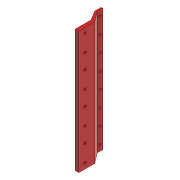
# Autodesk Inventor part: intake guide mount
Saved by Autodesk Inventor 2020 (Build 240168000, 168)
## iProperties
Created: 2020-02-10
Part Number: intake guide mount
Material: Generic
Document SubType Name: Modeling
Designer: ball
Density: 1 g/cm^3
Appearance: Default
Author: ball
Autodesk Inventor part; units mm, degrees
ref_plane "YZ Plane" through (0, 0, 0) normal (1, 0, 0) x (0, 1, 0)
ref_plane "XZ Plane" through (0, 0, 0) normal (0, 1, 0) x (-1, 0, 0)
ref_plane "XY Plane" through (0, 0, 0) normal (0, 0, 1) x (1, 0, 0)
sketch "Sketch1" plane through (0, 0, 0) normal (0, 1, 0) x (-1, 0, 0)
  line L0 (0, 0) -> (-19.05, 0) construction
  line L1 (-19.05, 0) -> (-19.05, -19.05) construction
  line L2 (-19.05, -19.05) -> (0, -19.05) construction
  line L3 (0, -19.05) -> (0, 0) construction
  line L4 (0, 0) -> (279.4, 0) construction
  line L5 (279.4, 0) -> (279.4, -35.5) construction
  line L6 (279.4, -35.5) -> (0, -35.5) construction
  line L7 (0, -35.5) -> (0, 0) construction
  line L8 (-47.8536, 0) -> (-47.8536, -76.2) construction
  line L9 (-19.05, 0) -> (-24.9936, 0)
  line L10 (-24.9936, 0) -> (-24.9936, -25.4)
  line L11 (-24.9936, -25.4) -> (-19.05, -25.4)
  line L12 (-19.05, -25.4) -> (-19.05, 0)
  line L13 (-9.7536, -51) -> (-12.2936, -51)
  line L14 (-12.2936, -51) -> (-12.2936, -42.11)
  line L15 (-9.7536, -40.84) -> (-9.7536, -51)
  line L16 (-9.7536, -40.84) -> (-19.05, -25.4)
  line L17 (-9.7536, -42.11) -> (-12.2936, -42.11) construction
  line L18 (-12.2936, -42.11) -> (-24.9936, -25.4)
  dimension "d0" = 19.05
  dimension "d1" = 19.05
  dimension "d2" = 279.4
  dimension "d3" = 35.5
  dimension "d4" = 76.2
  dimension "d5" = 28.8036
  dimension "d6" = 38.1
  dimension "d7" = 51
  dimension "d8" = 5.9436
  dimension "d9" = 25.4
  dimension "d12" = 8.89
  constraints: 38 end point, 7 parallel, 5 perpendicular, 4 horizontal, 1 point on line, 1 vertical
  measures "d0" distance of L2.end L1.end
  measures "d1" distance of L1.end L0.end
  measures "d2" distance of L5.end L6.end
  measures "d3" distance of L4.end L5.end
  measures "d4" distance of L8.start L8.end
  measures "d5" distance between parallel lines of L1 L8
  measures "d6" distance from line of L8 L13.start
  measures "d7" distance from line of L4 L13.start
  measures "d8" distance of L11.end L10.end
  measures "d9" distance of L10.end L9.end
  measures "d12" distance between parallel lines of L13 L17
extrude "Extrusion1" add sketch "Sketch1" along normal blind 195.58
sketch "Sketch2" plane through (24.9936, 0, 0) normal (1, 0, 0) x (0, 0, -1)
  circle A0 centre (9.525, 8.89) radius 1.9304
  circle A1 centre (9.525, 35.8394) radius 1.9304
  line L0 (0, 0) -> (25.4, 0) projected
  line L1 (0, 0) -> (0, 195.58) projected
  circle A2 centre (9.525, 86.6394) radius 1.9304
  circle A3 centre (9.525, 59.69) radius 1.9304
  circle A4 centre (9.525, 137.4394) radius 1.9304
  circle A5 centre (9.525, 110.49) radius 1.9304
  circle A6 centre (9.525, 188.2394) radius 1.9304
  circle A7 centre (9.525, 161.29) radius 1.9304
  dimension "d16" = 3.8608
  dimension "d17" = 3.8608
  dimension "d18" = 26.9494
  dimension "d19" = 8.89
  dimension "d20" = 9.525
  dimension "d21" = 9.525
  dimension "d24" = 50.8
  constraints: 8 centre point, 1 vertical, 12 other
  measures "d16" diameter of A0
  measures "d17" diameter of A1
  measures "d18" distance of A0.centre A1.centre
  measures "d19" distance from line of L0 A0.centre
  measures "d20" distance from line of L1 A0.centre
  measures "d21" distance from line of L1 A1.centre
  measures "d24" distance of A1.centre A2.centre
extrude "Extrusion2" cut sketch "Sketch2" against normal blind 195.58
sketch "Sketch3" plane through (9.7536, 0, -51) normal (-1, 0, 0) x (0, 0, 1)
  circle A0 centre (4.445, 8.89) radius 1.9304
  line L0 (0, 0) -> (0, 195.58) projected
  line L1 (0, 0) -> (10.16, 0) projected
  circle A1 centre (4.445, 34.29) radius 1.9304
  circle A2 centre (4.445, 59.69) radius 1.9304
  circle A3 centre (4.445, 85.09) radius 1.9304
  circle A4 centre (4.445, 110.49) radius 1.9304
  circle A5 centre (4.445, 135.89) radius 1.9304
  circle A6 centre (4.445, 161.29) radius 1.9304
  circle A7 centre (4.445, 186.69) radius 1.9304
  point P0 (51, 0)
  dimension "d31" = 3.8608
  dimension "d32" = 4.445
  dimension "d33" = 8.89
  dimension "d36" = 25.4
  constraints: 8 centre point, 1 vertical, 14 other
  measures "d31" diameter of A0
  measures "d32" distance from line of A0.centre L0
  measures "d33" distance from line of L1 A0.centre
  measures "d36" distance of A0.centre A1.centre
extrude "Extrusion3" cut sketch "Sketch3" against normal through all
equation "\"d21\" = d20"
body "Solid1"
